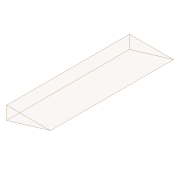
# Autodesk Inventor part: ramp
Saved by Autodesk Inventor 2019 (Build 230136000, 136)
## iProperties
Created: 2023-10-12
Part Number: ramp
Material: PMMA Plastic
Document SubType Name: Modeling
Designer: prich
Density: 1.188 g/cm^3
Appearance: Polycarbonate - Clear
Mass: 0.127885 g
Surface Area: 2.76978 cm^2
Volume: 0.107648 cm^3
Author: prich
Autodesk Inventor part; units mm, degrees
ref_plane "YZ Plane" through (0, 0, 0) normal (1, 0, 0) x (0, 1, 0)
ref_plane "XZ Plane" through (0, 0, 0) normal (0, 1, 0) x (-1, 0, 0)
ref_plane "XY Plane" through (0, 0, 0) normal (0, 0, 1) x (1, 0, 0)
sketch "Sketch1" plane through (0, 0, 0) normal (0, 0, 1) x (1, 0, 0)
  line L0 (0, 0) -> (6.3563, 0)
  line L1 (6.3563, 0) -> (0, -1.905)
  line L2 (0, -1.905) -> (0, 0)
  dimension "d0" = 6.3563
  dimension "d1" = 1.905
  constraints: 6 end point, 1 horizontal, 1 perpendicular
  measures "d0" distance of L0.start L0.end
  measures "d1" distance of L1.end L0.start
extrude "Extrusion1" add sketch "Sketch1" along normal blind 17.78
body "Solid1"
